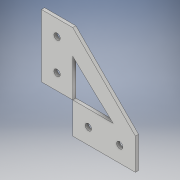
# Autodesk Inventor part: special brace
Saved by Autodesk Inventor 2018 (Build 220112000, 112)
## iProperties
Created: 2018-12-12
Part Number: special brace
Material: Generic
Document SubType Name: Modeling
Designer: s-4008082
Density: 1 g/cm^3
Appearance: Default
Author: s-4008082
Autodesk Inventor part; units mm, degrees
ref_plane "YZ Plane" through (0, 0, 0) normal (1, 0, 0) x (0, 1, 0)
ref_plane "XZ Plane" through (0, 0, 0) normal (0, 1, 0) x (-1, 0, 0)
ref_plane "XY Plane" through (0, 0, 0) normal (0, 0, 1) x (1, 0, 0)
sketch "Sketch1" plane through (0, 0, 0) normal (0, 0, 1) x (1, 0, 0)
  line L0 (0, 0) -> (25.4, 0)
  line L1 (25.4, 0) -> (25.4, 50.8)
  line L2 (25.4, 50.8) -> (0, 50.8)
  line L3 (0, 50.8) -> (0, 0)
  line L4 (25.4, 0) -> (76.2, 0)
  line L5 (76.2, 0) -> (76.2, -25.4)
  line L6 (76.2, -25.4) -> (25.4, -25.4)
  line L7 (25.4, -25.4) -> (25.4, 0)
  line L8 (76.2, 0) -> (25.4, 50.8)
  line L9 (25.4, 30.6304) -> (58.0931, 0)
  dimension "d0" = 25.4
  dimension "d1" = 50.8
  dimension "d2" = 50.8
  dimension "d3" = 25.4
  dimension "d4" = 1.866
  constraints: 20 end point, 4 parallel, 2 horizontal, 2 perpendicular, 2 point on line
  measures "d0" distance of L1.end L2.end
  measures "d1" distance of L0.end L1.end
  measures "d2" distance of L5.end L6.end
  measures "d3" distance of L4.end L5.end
  measures "d4" angle of L9 L8
extrude "Extrusion1" add sketch "Sketch1" along normal blind 2.54 contours L3 L2 L1 L0 | L4 L5 L6 L7 | L1 L8 L4 L9
sketch "Sketch2" plane through (0, 0, 2.54) normal (0, 0, 1) x (1, 0, 0)
  circle A0 centre (12.7, 12.7) radius 2.5797
  line L0 (0, 50.8) -> (0, 0) projected
  line L1 (0, 0) -> (25.4, 0) projected
  circle A1 centre (12.7, 38.1) radius 2.5797
  line L2 (25.4, 50.8) -> (0, 50.8) projected
  circle A2 centre (38.1, -12.7) radius 2.5797
  circle A3 centre (63.5, -12.7) radius 2.5797
  line L3 (25.4, 0) -> (25.4, -25.4) projected
  line L4 (25.4, -25.4) -> (76.2, -25.4) projected
  line L5 (76.2, -25.4) -> (76.2, 0) projected
  dimension "d7" = 12.7
  dimension "d8" = 12.7
  dimension "d9" = 5.1594
  dimension "d10" = 12.7
  dimension "d11" = 5.1594
  dimension "d12" = 25.4
  dimension "d13" = 12.7
  dimension "d14" = 12.7
  dimension "d15" = 12.7
  dimension "d16" = 12.7
  dimension "d17" = 5.1594
  dimension "d18" = 5.1594
  constraints: 4 centre point
  measures "d7" distance from line of L0 A0.centre
  measures "d8" distance from line of L1 A0.centre
  measures "d9" diameter of A0
  measures "d10" distance from line of L2 A1.centre
  measures "d11" diameter of A1
  measures "d12" distance of A0.centre A1.centre
  measures "d13" distance from line of L3 A2.centre
  measures "d14" distance from line of L4 A2.centre
  measures "d15" distance from line of L5 A3.centre
  measures "d16" distance from line of L4 A3.centre
  measures "d17" diameter of A2
  measures "d18" diameter of A3
extrude "Extrusion2" cut sketch "Sketch2" against normal blind 2.54
body "Solid1"
